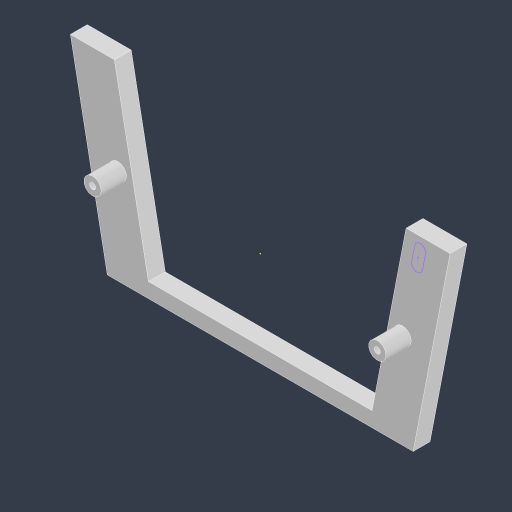
# Autodesk Inventor part: Touchpad Top
Saved by Autodesk Inventor 2023.4 (Build 274418000, 418)
## iProperties
Created: 2024-02-23
Part Number: Touchpad Top
Material: Generic
Document SubType Name: Modeling
Designer: JoaoSilva
Density: 1 g/cm^3
Appearance: Default
Author: JoaoSilva
Autodesk Inventor part; units mm, degrees
ref_plane "YZ Plane" through (0, 0, 0) normal (1, 0, 0) x (0, 1, 0)
ref_plane "XZ Plane" through (0, 0, 0) normal (0, 1, 0) x (-1, 0, 0)
ref_plane "XY Plane" through (0, 0, 0) normal (0, 0, 1) x (1, 0, 0)
sketch "Sketch1" plane through (0, 0, 0) normal (0, 0, 1) x (1, 0, 0)
  line L0 (-36.2529, -22.5) -> (36.2529, -22.5)
  line L1 (36.2529, -22.5) -> (45, 22.5)
  line L2 (45, 22.5) -> (-45, 22.5)
  line L3 (-45, 22.5) -> (-36.2529, -22.5)
  point P0 (0, 0)
  point P1 (0, -22.5)
  point P2 (40.6264, 0)
  point P3 (0, 22.5)
  dimension "d0" = 45
  dimension "d1" = 22
  dimension "d2" = 90
  constraints: 8 end point, 3 midpoint, 2 vertical alignment, 1 equal length, 1 horizontal, 1 horizontal alignment, 1 parallel
  measures "d0" distance between parallel lines of L2 L0
  measures "d1" angle of L3 L1
  measures "d2" distance of L1.end L2.end
extrude "Extrusion1" add sketch "Sketch1" along normal blind 4
sketch "Sketch2" plane through (0, 0, 4) normal (0, 0, 1) x (1, 0, 0)
  line L0 (-33.75, 0) -> (33.75, 0) construction
  circle A0 centre (33.75, 0) radius 2.05
  circle A1 centre (-33.75, 0) radius 2.05
  line L1 (45, 22.5) -> (-45, 22.5) projected
  line L2 (-36.2529, -22.5) -> (36.2529, -22.5) projected
  circle A2 centre (33.75, 0) radius 0.75
  circle A3 centre (-33.75, 0) radius 0.75
  point P0 (0, 0)
  point P1 (0, 0)
  dimension "d5" = 67.5
  dimension "d6" = 4.1
  dimension "d7" = 22.5
  dimension "d8" = 45
  dimension "d9" = 1.5
  constraints: 5 coincident, 4 centre point, 2 end point, 2 equal radius, 1 horizontal, 1 midpoint
  measures "d5" distance of L0.start L0.end
  measures "d6" diameter of A0
  measures "d7" distance between parallel lines of L1 L0
  measures "d8" distance between parallel lines of L1 L2
  measures "d9" diameter of A2
extrude "Extrusion2" add sketch "Sketch2" along normal blind 6
sketch "Sketch3" plane through (0, 0, 4) normal (0, 0, 1) x (1, 0, 0)
  line L0 (-26.5068, -19) -> (26.5068, -19)
  line L1 (26.5068, -19) -> (34.5736, 22.5)
  line L2 (34.5736, 22.5) -> (-34.5736, 22.5)
  line L3 (-34.5736, 22.5) -> (-26.5068, -19)
  line L4 (-45, 22.5) -> (-36.2529, -22.5) projected
  line L5 (36.2529, -22.5) -> (45, 22.5) projected
  line L6 (-30.2, 0) -> (30.2, 0) construction
  circle A0 centre (33.75, 0) radius 2.05 projected
  line L7 (45, 22.5) -> (-45, 22.5) projected
  circle A1 centre (33.75, 0) radius 0.75 projected
  point P0 (0, 0)
  point P1 (0, -19)
  dimension "d13" = 60.4
  dimension "d14" = 19
  constraints: 10 end point, 3 parallel, 3 point on line, 2 horizontal, 1 collinear, 1 midpoint, 1 vertical alignment
  measures "d13" distance of L6.start L6.end
  measures "d14" distance from line of A1.centre L0
extrude "Extrusion3" cut sketch "Sketch3" against normal through all contours L3 L2 L1 L0
sketch "Sketch4" plane through (0, 0, 4) normal (0, 0, 1) x (1, 0, 0)
  line L0 (37.1379, 16.0576) -> (37.8822, 19.7792) construction
  line L1 (35.8639, 16.3124) -> (36.6083, 20.034)
  line L2 (39.1561, 19.5244) -> (38.4118, 15.8028)
  arc A0 (35.8639, 16.3124) -> (38.4118, 15.8028) centre (37.1379, 16.0576) ccw
  arc A1 (39.1561, 19.5244) -> (36.6083, 20.034) centre (37.8822, 19.7792) ccw
  point P0 (0, 0)
  point P1 (37.51, 17.9184)
  constraints: 8 end point, 4 point on circle, 4 tangent, 2 centre point, 1 midpoint, 1 parallel
equation "\"d7\" = 0.5 * d8"
body "Solid1"
